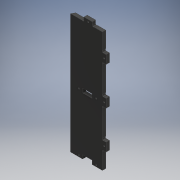
# Autodesk Inventor part: BA03
Saved by Autodesk Inventor 2017 (Build 210142000, 142)
## iProperties
Created: 2019-05-22
Part Number: BA03
Material: Wood (Cherry)
Document SubType Name: Modeling
Designer: Dell
Density: 0.63 g/cm^3
Appearance: Smooth - Black
Mass: 235.193 g
Surface Area: 754.585 cm^2
Volume: 373.322 cm^3
Author: Dell
Autodesk Inventor part; units mm, degrees
ref_plane "YZ Plane" through (0, 0, 0) normal (1, 0, 0) x (0, 1, 0)
ref_plane "XZ Plane" through (0, 0, 0) normal (0, 1, 0) x (-1, 0, 0)
ref_plane "XY Plane" through (0, 0, 0) normal (0, 0, 1) x (1, 0, 0)
sketch "Sketch1" plane through (0, 0, 0) normal (0, 0, 1) x (1, 0, 0)
  line L0 (0, 0) -> (92.075, 0)
  line L1 (92.075, 0) -> (92.075, 9.525)
  line L2 (92.075, 9.525) -> (5.4993, 9.525)
  line L3 (5.4993, 9.525) -> (0, 0)
  dimension "d0" = 92.075
  dimension "d1" = 9.525
  dimension "d2" = 60
  constraints: 8 end point, 2 perpendicular, 1 horizontal
  measures "d0" distance of L0.start L0.end
  measures "d1" distance of L0.end L1.end
  measures "d2" angle of L0 L3
extrude "Extrusion1" add sketch "Sketch1" along normal blind 346.075
sketch "Sketch2" plane through (0, 0, 0) normal (0, -1, 0) x (1, 0, 0)
  line L0 (38.1, 346.075) -> (63.5, 346.075)
  line L1 (63.5, 346.075) -> (63.5, 355.6)
  line L2 (63.5, 355.6) -> (38.1, 355.6)
  line L3 (38.1, 355.6) -> (38.1, 346.075)
  line L4 (0, 346.075) -> (101.6, 346.075)
  line L5 (0, 346.075) -> (92.075, 346.075) projected
  point P0 (0, 0)
  point P1 (50.8, 346.075)
  dimension "d5" = 25.4
  dimension "d6" = 9.525
  dimension "d9" = 101.6
  constraints: 10 end point, 2 midpoint, 2 parallel, 1 collinear, 1 horizontal, 1 perpendicular
  measures "d5" distance of L2.end L1.end
  measures "d6" distance of L1.end L0.end
  measures "d9" distance of L4.start L4.end
extrude "Extrusion2" add sketch "Sketch2" against normal blind 9.525
sketch "Sketch3" plane through (0, 0, 0) normal (0, -1, 0) x (1, 0, 0)
  line L0 (63.5, 346.075) -> (63.5, 355.6) projected
  line L1 (63.5, 355.6) -> (38.1, 355.6) projected
  circle A0 centre (50.8, 350.8375) radius 2.25
  point P0 (0, 0)
  point P1 (50.8, 355.6)
  point P2 (63.5, 350.8375)
  dimension "d10" = 4.5
  constraints: 2 midpoint, 1 centre point, 1 horizontal alignment, 1 vertical alignment
  measures "d10" diameter of A0
extrude "Extrusion3" cut sketch "Sketch3" against normal through all
sketch "Sketch4" plane through (0, 0, 0) normal (0, -1, 0) x (1, 0, 0)
  line L0 (92.075, 0) -> (92.075, 346.075) projected
  line L1 (92.075, 50.8) -> (101.6, 50.8)
  line L2 (101.6, 50.8) -> (101.6, 76.2)
  line L3 (101.6, 76.2) -> (92.075, 76.2)
  line L4 (92.075, 76.2) -> (92.075, 50.8)
  line L5 (92.075, 295.275) -> (101.6, 295.275)
  line L6 (101.6, 295.275) -> (101.6, 269.875)
  line L7 (101.6, 269.875) -> (92.075, 269.875)
  line L8 (92.075, 269.875) -> (92.075, 295.275)
  line L9 (92.075, 185.7375) -> (101.6, 185.7375)
  line L10 (101.6, 185.7375) -> (101.6, 160.3375)
  line L11 (101.6, 160.3375) -> (92.075, 160.3375)
  line L12 (92.075, 160.3375) -> (92.075, 185.7375)
  circle A0 centre (96.8375, 282.575) radius 2.25
  circle A1 centre (96.8375, 173.0375) radius 2.25
  circle A2 centre (96.8375, 63.5) radius 2.25
  point P0 (0, 0)
  point P1 (92.075, 173.0375)
  point P2 (96.8375, 295.275)
  point P3 (96.8375, 185.7375)
  point P4 (96.8375, 76.2)
  point P5 (101.6, 282.575)
  point P6 (101.6, 173.0375)
  point P7 (101.6, 63.5)
  dimension "d14" = 25.4
  dimension "d15" = 9.525
  dimension "d16" = 25.4
  dimension "d18" = 25.4
  dimension "d19" = 50.8
  dimension "d20" = 50.8
  dimension "d21" = 4.5
  dimension "d22" = 4.5
  dimension "d23" = 4.5
  constraints: 24 end point, 8 midpoint, 6 parallel, 5 vertical alignment, 3 centre point, 3 horizontal, 3 horizontal alignment, 3 perpendicular, 3 point on line
  measures "d14" distance of L2.end L1.end
  measures "d15" distance of L6.end L7.end
  measures "d16" distance of L5.end L6.end
  measures "d18" distance of L9.end L10.end
  measures "d19" distance from line of L0.end L5
  measures "d20" distance from line of L0.start L1
  measures "d21" diameter of A0
  measures "d22" diameter of A1
  measures "d23" diameter of A2
extrude "Extrusion4" add sketch "Sketch4" against normal blind 9.525
sketch "Sketch6" plane through (92.075, 0, 295.275) normal (0, 0, 1) x (1, 0, 0)
  line L0 (-92.075, 0) -> (-75.5772, 9.525)
  line L1 (0, 9.525) -> (-86.5757, 9.525) projected
  line L2 (-92.075, 0) -> (0, 0) projected
  line L3 (-75.5772, 9.525) -> (-75.5772, 0)
  line L4 (-86.5757, 9.525) -> (-92.075, 0) projected
  line L5 (-81.0765, 6.35) -> (-81.0765, 9.525)
  line L6 (-81.0765, 9.525) -> (-86.5757, 9.525)
  dimension "d28" = 30
  dimension "d31" = 12.7
  constraints: 8 end point, 4 point on line, 1 collinear, 1 perpendicular, 1 vertical
  measures "d28" angle of L0 L2
  measures "d31" distance of L0.start L5.start
extrude "Extrusion6" [suppressed]
sketch "Sketch7" plane through (92.075, 0, 185.7375) normal (0, 0, 1) x (1, 0, 0)
  line L0 (-77.9015, 12.7) -> (-77.9015, 6.35) projected
  line L1 (-81.5677, 12.7) -> (-77.9015, 12.7) projected
  line L2 (-88.9, 0) -> (-81.5677, 12.7) projected
  line L3 (-77.9015, 6.35) -> (-88.9, 0) projected
  point P0 (-92.075, 0)
extrude "Extrusion7" [suppressed]
sketch "Sketch8" plane through (92.075, 0, 76.2) normal (0, 0, 1) x (1, 0, 0)
  line L0 (-77.9015, 12.7) -> (-77.9015, 6.35) projected
  line L1 (-81.5677, 12.7) -> (-77.9015, 12.7) projected
  line L2 (-88.9, 0) -> (-81.5677, 12.7) projected
  line L3 (-77.9015, 6.35) -> (-88.9, 0) projected
  point P0 (-92.075, 0)
extrude "Extrusion8" [suppressed]
sketch "Sketch10" plane through (5.4993, 9.525, 0) normal (0, 1, 0) x (1, 0, 0)
  circle A0 centre (18.2879, -4.7625) radius 2.25
  line L0 (85.64, -9.525) -> (0.9358, -9.525)
  circle A1 centre (68.2879, -4.7625) radius 2.25
  line L1 (30.5879, -9.525) -> (55.9879, -9.525)
  line L2 (55.9879, -9.525) -> (55.9879, 0)
  line L3 (55.9879, 0) -> (30.5879, 0)
  line L4 (30.5879, 0) -> (30.5879, -9.525)
  line L5 (18.2879, -4.7625) -> (68.2879, -4.7625) construction
  line L6 (86.5757, 0) -> (0, 0) projected
  point P0 (-5.4993, 0)
  point P1 (43.2879, -4.7625)
  point P2 (43.2879, -9.525)
  point P3 (43.2879, -9.525)
  point P4 (43.2879, 0)
  point P5 (30.5879, -4.7625)
  dimension "d39" = 4.5
  dimension "d41" = 4.5
  dimension "d42" = 25.4
  dimension "d43" = 9.525
  dimension "d44" = 50
  constraints: 12 end point, 8 midpoint, 3 horizontal, 2 centre point, 2 parallel, 1 horizontal alignment, 1 perpendicular, 1 point on line, 1 vertical alignment
  measures "d39" diameter of A0
  measures "d41" diameter of A1
  measures "d42" distance of L3.end L2.end
  measures "d43" distance of L2.end L1.end
  measures "d44" distance of L5.start L5.end
extrude "Extrusion10" cut sketch "Sketch10" against normal through all
sketch "Sketch11" plane through (38.1, 0, 355.6) normal (0, -1, 0) x (1, 0, 0)
  line L0 (23.3871, -189.3875) -> (-2.0129, -189.3875)
  line L1 (-2.0129, -189.3875) -> (-2.0129, -179.8625)
  line L2 (-2.0129, -179.8625) -> (23.3871, -179.8625)
  line L3 (23.3871, -179.8625) -> (23.3871, -189.3875)
  line L4 (63.5, -169.8625) -> (53.975, -169.8625) projected
  line L5 (-2.0129, -346.075) -> (23.3871, -346.075) projected
  point P0 (-38.1, -355.6)
  point P1 (10.6871, -189.3875)
  point P2 (10.6871, -346.075)
  dimension "d47" = 25.4
  dimension "d48" = 9.525
  dimension "d85" = 10
  constraints: 8 end point, 2 midpoint, 2 parallel, 1 horizontal, 1 perpendicular, 1 vertical alignment
  measures "d47" distance of L1.end L2.end
  measures "d48" distance of L0.end L1.end
  measures "d85" vertical distance of L2.end L4.start
extrude "Extrusion11" cut sketch "Sketch11" against normal through all
sketch "Sketch12" plane through (38.1, 0, 355.6) normal (0, -1, 0) x (1, 0, 0)
  circle A0 centre (-14.3129, -184.625) radius 2.25
  circle A1 centre (35.6871, -184.625) radius 2.25
  circle A2 centre (-14.3129, -350.8375) radius 2.25 projected
  circle A3 centre (35.6871, -350.8375) radius 2.25 projected
  line L0 (23.3871, -179.8625) -> (23.3871, -189.3875) projected
  point P0 (-38.1, -355.6)
  point P1 (23.3871, -184.625)
  dimension "d52" = 4.5
  dimension "d53" = 4.5
  constraints: 2 centre point, 2 horizontal alignment, 2 vertical alignment, 1 midpoint
  measures "d52" diameter of A0
  measures "d53" diameter of A1
extrude "Extrusion12" cut sketch "Sketch12" against normal through all contours A0 | A1
sketch "Sketch13" plane through (5.4993, 9.525, 346.075) normal (0, 1, 0) x (1, 0, 0)
  line L0 (55.9879, 346.075) -> (86.5757, 346.075) projected
  line L1 (57.2579, 346.075) -> (29.3179, 346.075)
  line L2 (29.3179, 346.075) -> (29.3179, 335.28)
  line L3 (29.3179, 335.28) -> (57.2579, 335.28)
  line L4 (57.2579, 335.28) -> (57.2579, 346.075)
  line L5 (57.2579, 181.1325) -> (29.3179, 181.1325)
  line L6 (29.3179, 181.1325) -> (29.3179, 169.0675)
  line L7 (29.3179, 169.0675) -> (57.2579, 169.0675)
  line L8 (57.2579, 169.0675) -> (57.2579, 181.1325)
  line L9 (55.9879, 336.55) -> (30.5879, 336.55) projected
  line L10 (30.5879, 179.8625) -> (55.9879, 179.8625) projected
  line L11 (55.9879, 179.8625) -> (55.9879, 170.3375) projected
  circle A0 centre (60.2458, -2.2451) radius 3.175
  circle A1 centre (30.3557, -2.2451) radius 3.175
  circle A2 centre (88.8208, 48.5549) radius 3.175
  circle A3 centre (88.8208, 78.4451) radius 3.175
  circle A4 centre (88.8208, 158.0924) radius 3.175
  circle A5 centre (88.8208, 187.9826) radius 3.175
  circle A6 centre (88.8208, 267.6299) radius 3.175
  circle A7 centre (88.8208, 297.5201) radius 3.175
  line L12 (96.1007, 295.275) -> (86.5757, 295.275) projected
  line L13 (86.5757, 295.275) -> (88.8208, 297.5201)
  line L14 (60.2458, -2.2451) -> (58.0007, 0) construction
  line L15 (58.0007, -9.525) -> (58.0007, 0) projected
  point P0 (-5.4993, 346.075)
  point P1 (43.2879, 336.55)
  point P2 (43.2879, 335.28)
  point P3 (43.2879, 179.8625)
  point P4 (43.2879, 181.1325)
  point P5 (55.9879, 175.1)
  point P6 (57.2579, 175.1)
  point P7 (86.5757, 269.875)
  point P8 (86.5757, 185.7375)
  point P9 (86.5757, 160.3375)
  point P10 (86.5757, 50.8)
  point P11 (86.5757, 76.2)
  point P12 (32.6007, 0)
  dimension "d61" = 6.35
  dimension "d62" = 6.35
  dimension "d63" = 6.35
  dimension "d64" = 6.35
  dimension "d65" = 6.35
  dimension "d66" = 6.35
  dimension "d67" = 6.35
  dimension "d68" = 6.35
  dimension "d56" = 1.27
  dimension "d57" = 1.27
  dimension "d58" = 1.27
  dimension "d69" = 45
  dimension "d70" = 45
  constraints: 20 end point, 9 vertical alignment, 6 midpoint, 4 parallel, 3 point on line, 2 horizontal, 2 horizontal alignment, 2 perpendicular, 1 coincident, 24 other
  measures "d56" distance between parallel lines of L3 L9
  measures "d57" distance between parallel lines of L8 L11
  measures "d58" distance between parallel lines of L5 L10
  measures "d69" angle of L12 L13
  measures "d70" angle of L15 L14
extrude "Extrusion13" cut sketch "Sketch13" against normal through all
sketch "Sketch14" plane through (5.4993, 9.525, 346.075) normal (0, 1, 0) x (1, 0, 0)
  line L0 (96.1007, 50.8) -> (91.0659, 50.8) projected
  line L1 (96.1007, 50.8) -> (90.1572, 50.8)
  line L2 (90.1572, 50.8) -> (90.1572, 51.435)
  line L3 (90.1572, 51.435) -> (96.1007, 51.435)
  line L4 (96.1007, 51.435) -> (96.1007, 50.8)
  line L5 (96.1007, 50.8) -> (96.1007, 76.2) projected
  line L6 (96.1007, 76.2) -> (90.1572, 76.2)
  line L7 (90.1572, 76.2) -> (90.1572, 75.565)
  line L8 (90.1572, 75.565) -> (96.1007, 75.565)
  line L9 (96.1007, 75.565) -> (96.1007, 76.2)
  line L10 (96.1007, 160.3375) -> (91.0659, 160.3375) projected
  line L11 (96.1007, 160.3375) -> (90.1572, 160.3375)
  line L12 (90.1572, 160.3375) -> (90.1572, 160.9725)
  line L13 (90.1572, 160.9725) -> (96.1007, 160.9725)
  line L14 (96.1007, 160.9725) -> (96.1007, 160.3375)
  line L15 (91.0659, 185.7375) -> (96.1007, 185.7375) projected
  line L16 (96.1007, 185.7375) -> (90.1572, 185.7375)
  line L17 (90.1572, 185.7375) -> (90.1572, 185.1025)
  line L18 (90.1572, 185.1025) -> (96.1007, 185.1025)
  line L19 (96.1007, 185.1025) -> (96.1007, 185.7375)
  line L20 (96.1007, 269.875) -> (96.1007, 295.275) projected
  line L21 (96.1007, 269.875) -> (90.1572, 269.875)
  line L22 (90.1572, 269.875) -> (90.1572, 270.51)
  line L23 (90.1572, 270.51) -> (96.1007, 270.51)
  line L24 (96.1007, 270.51) -> (96.1007, 269.875)
  line L25 (96.1007, 295.275) -> (90.1572, 295.275)
  line L26 (90.1572, 295.275) -> (90.1572, 294.64)
  line L27 (90.1572, 294.64) -> (96.1007, 294.64)
  line L28 (96.1007, 294.64) -> (96.1007, 295.275)
  arc A0 (86.5757, 299.7651) -> (91.0659, 295.275) centre (88.8208, 297.5201) ccw projected
  line L29 (32.6007, -9.525) -> (58.0007, -9.525) projected
  arc A1 (62.4909, 0) -> (58.0007, -4.4901) centre (60.2458, -2.2451) ccw projected
  line L30 (58.0007, -9.525) -> (57.3657, -9.525)
  line L31 (57.3657, -9.525) -> (57.3657, -3.5814)
  line L32 (57.3657, -3.5814) -> (58.0007, -3.5814)
  line L33 (58.0007, -3.5814) -> (58.0007, -9.525)
  line L34 (32.6007, -4.4901) -> (32.6007, -9.525) projected
  arc A2 (32.6007, -4.4901) -> (28.1106, 0) centre (30.3557, -2.2451) ccw projected
  line L35 (32.6007, -9.525) -> (33.2357, -9.525)
  line L36 (33.2357, -9.525) -> (33.2357, -3.5814)
  line L37 (33.2357, -3.5814) -> (32.6007, -3.5814)
  line L38 (32.6007, -3.5814) -> (32.6007, -9.525)
  point P0 (-5.4993, 346.075)
  dimension "d71" = 0.635
  dimension "d72" = 0.635
  dimension "d73" = 0.635
  dimension "d74" = 0.635
  dimension "d75" = 0.635
  dimension "d76" = 0.635
  dimension "d77" = 0.635
  constraints: 64 end point, 16 parallel, 8 horizontal, 8 perpendicular, 5 point on line, 3 point on circle, 1 vertical alignment
  measures "d71" distance between parallel lines of L25 L27
  measures "d72" distance between parallel lines of L21 L23
  measures "d73" distance between parallel lines of L16 L18
  measures "d74" distance between parallel lines of L11 L13
  measures "d75" distance between parallel lines of L0 L3
  measures "d76" distance between parallel lines of L6 L8
  measures "d77" distance between parallel lines of L33 L31
extrude "Extrusion14" cut sketch "Sketch14" against normal through all
sketch "Sketch15" plane through (5.4993, 9.525, 346.075) normal (0, 1, 0) x (1, 0, 0)
  line L0 (96.1007, 270.51) -> (90.1572, 270.51) projected
  line L1 (96.1007, 270.51) -> (97.3707, 270.51)
  line L2 (97.3707, 270.51) -> (97.3707, 294.64)
  line L3 (97.3707, 294.64) -> (96.1007, 294.64)
  line L4 (96.1007, 294.64) -> (96.1007, 270.51)
  line L5 (96.1007, 185.1025) -> (97.3707, 185.1025)
  line L6 (97.3707, 185.1025) -> (97.3707, 160.9725)
  line L7 (97.3707, 160.9725) -> (96.1007, 160.9725)
  line L8 (96.1007, 160.9725) -> (96.1007, 185.1025)
  line L9 (96.1007, 51.435) -> (96.1007, 75.565) projected
  line L10 (96.1007, 75.565) -> (97.3707, 75.565)
  line L11 (97.3707, 75.565) -> (97.3707, 51.435)
  line L12 (97.3707, 51.435) -> (96.1007, 51.435)
  line L13 (96.1007, 51.435) -> (96.1007, 75.565)
  line L14 (33.2357, -9.525) -> (57.3657, -9.525) projected
  line L15 (57.3657, -9.525) -> (33.2357, -9.525)
  line L16 (33.2357, -9.525) -> (33.2357, -10.795)
  line L17 (33.2357, -10.795) -> (57.3657, -10.795)
  line L18 (57.3657, -10.795) -> (57.3657, -9.525)
  point P0 (-5.4993, 346.075)
  dimension "d80" = 1.27
  dimension "d81" = 1.27
  constraints: 32 end point, 8 parallel, 4 horizontal, 4 perpendicular, 3 coincident, 2 point on line, 1 vertical alignment
  measures "d80" distance of L2.end point (96.101, 294.64)
  measures "d81" distance of L17.end L14.end
extrude "Extrusion15" add sketch "Sketch15" against normal blind 9.525
equation "\"d1\" = Panel_Thickness"
equation "\"d6\" = Panel_Thickness"
equation "\"d7\" = Panel_Thickness"
equation "\"d15\" = Panel_Thickness"
equation "\"d24\" = Panel_Thickness"
equation "\"d43\" = Panel_Thickness"
equation "\"d48\" = Panel_Thickness"
equation "\"d61\" = d63"
equation "\"d62\" = d61"
equation "\"d63\" = d65"
equation "\"d64\" = d65"
equation "\"d65\" = d68"
equation "\"d66\" = d68"
equation "\"d67\" = d68"
equation "\"d68\" = Tool_Dia"
equation "\"d56\" = Fit_Tolerance"
equation "\"d57\" = Fit_Tolerance"
equation "\"d58\" = Fit_Tolerance"
equation "\"d71\" = 0.5 * Fit_Tolerance"
equation "\"d72\" = 0.5 * Fit_Tolerance"
equation "\"d73\" = 0.5 * Fit_Tolerance"
equation "\"d74\" = 0.5 * Fit_Tolerance"
equation "\"d75\" = 0.5 * Fit_Tolerance"
equation "\"d76\" = 0.5 * Fit_Tolerance"
equation "\"d77\" = 0.5 * Fit_Tolerance"
equation "\"d80\" = Fit_Tolerance"
equation "\"d81\" = Fit_Tolerance"
equation "\"d82\" = Panel_Thickness"
equation "\"Panel_Thickness\" = 9.525"
equation "\"Fit_Tolerance\" = 1.27"
equation "\"Tool_Dia\" = 6.35"
body "Solid1"
